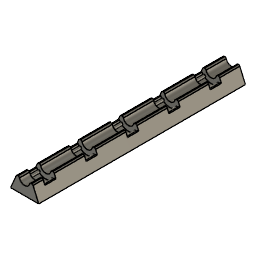
Frame_v1 (Autodesk Fusion 360 design; units mm, degrees)
Autodesk Fusion 360 part; units mm, degrees
sketch "Sketch1" plane through (0, 0, 0) normal (0, 1, 0) x (1, 0, 0)
  circle A0 centre (0, 0) radius 2.6
  line L0 (0, 0) -> (7, 0)
  line L1 (0, 0) -> (-7, 0)
  line L2 (7, 0) -> (7, 7)
  line L3 (7, 7) -> (-7, 7)
  line L4 (-7, 7) -> (-7, 0)
  line L5 (0, 0) -> (0, 7) construction
  circle A1 centre (0, 0) radius 5.1
  circle A2 centre (-3.4648, -3.4648) radius 0.75
  circle A3 centre (-3.4648, 3.4648) radius 0.75
  circle A4 centre (3.4648, 3.4648) radius 0.75
  circle A5 centre (3.4648, -3.4648) radius 0.75
  dimension "d1" = 5.2
  dimension "d2" = 7
  dimension "d3" = 7
  dimension "d4" = 10.2
  dimension "d10" = 1.5
  constraint coincident A0.centre L0.start
  constraint horizontal L0
  constraint parallel L0 L1
  constraint perpendicular L0 L2
  constraint perpendicular L2 L3
  constraint perpendicular L3 L4
  constraint midpoint L3 L5.end
  constraint perpendicular L3 L5
  constraint symmetric L0 L1 L5
  constraint concentric A0 A1
  measures "d1" diameter of A0
  measures "d2" distance of A0.centre L1.end
  measures "d3" distance of L1 L3
  measures "d4" diameter of A1
  measures "d10" diameter of A2
extrude "Extrude1" add sketch "Sketch1" along normal blind 20.5 contours A0 L0 L1 A1 A3 A4 | L0 L1 L2 L3 L4 A1 A3 A4 | A1 A4 | A1 A4 | A1 A3 | A1 A3 makes body 1
extrude "Extrude2" cut sketch "Sketch1" along normal blind 5.5 from surface at 5 contours A0 L0 L1 A1 A3 A4 bodies 1
move_face "OffsetFaces1" offset -0.1 2 faces at (-3.0183, 8.6667, -4.0674) (4.0674, 8.6667, -3.0183) on bodies 1
sketch "Sketch2" plane through (0, 0, 0) normal (0, 0, 1) x (1, 0, 0)
  line L0 (0, 0) -> (0, 250)
  constraint coincident L0.start origin
  constraint vertical L0
pattern_path "PathPattern1" count 5 spacing 20.5 from (0, 10.25, 0) path "Sketch2" along L0 of bodies 1 makes body 2 at (2.3333, 27.3333, -7) makes body 3 at (2.3333, 47.8333, -7) makes body 4 at (2.3333, 68.3333, -7) makes body 5 at (2.3333, 88.8333, -7)
combine "Combine1" operation add target body 5 tool bodies 4 2 3 1
chamfer "Chamfer1" distance 7 distance2 3 1 edges at (-7, 51.25, 0) measured on face at (-7, 68.3333, -2.3333) tangent chain off on bodies 5
chamfer "Chamfer2" distance 3 distance2 7 1 edges at (7, 51.25, 0) measured on face at (4.9, 99.1667, 0) tangent chain off on bodies 5
fillet "Fillet1" radius 0.75 24 edges at (-2.6, 97.5, 0) (-4, 97.5, 0) (2.6, 97.5, 0) (4, 97.5, 0) (2.6, 79.5, 0) (4, 79.5, 0) (-4, 79.5, 0) (-2.6, 79.5, 0) (-4, 59, 0) (-2.6, 59, 0) (2.6, 59, 0) (4, 59, 0) (4, 38.5, 0) (2.6, 38.5, 0) (-2.6, 38.5, 0) (-4, 38.5, 0) (-4, 18, 0) (-2.6, 18, 0) (2.6, 18, 0) (4, 18, 0) (-4, 2.5, 0) (-2.6, 2.5, 0) (2.6, 2.5, 0) (4, 2.5, 0) on bodies 5
fillet "Fillet2" radius 0.3 10 edges at (-4.7716, 7.75, -1.8005) (4.7716, 7.75, -1.8005) (-4.7716, 28.25, -1.8005) (4.7716, 28.25, -1.8005) (-4.7716, 48.75, -1.8005) (4.7716, 48.75, -1.8005) (-4.7716, 69.25, -1.8005) (4.7716, 69.25, -1.8005) (-4.7716, 89.75, -1.8005) (4.7716, 89.75, -1.8005) on bodies 5
